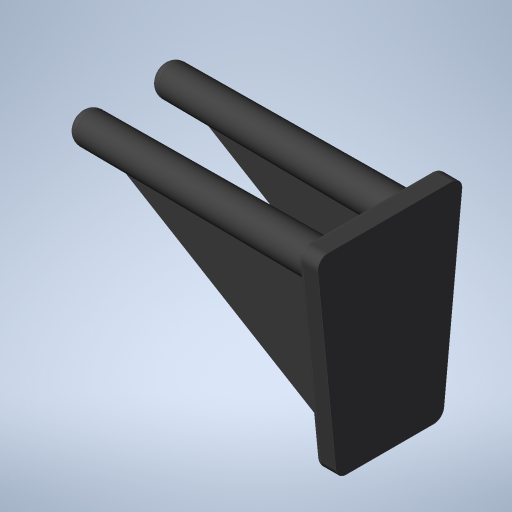
# Autodesk Inventor part: Ski Rack
Saved by Autodesk Inventor 2023 (Build 270158000, 158)
## iProperties
Created: 2022-12-21
Part Number: Ski Rack
Material: Generic
Document SubType Name: Modeling
Designer: tommy
Density: 1 g/cm^3
Appearance: Default
Author: tommy
Autodesk Inventor part; units mm, degrees
ref_plane "YZ Plane" through (0, 0, 0) normal (1, 0, 0) x (0, 1, 0)
ref_plane "XZ Plane" through (0, 0, 0) normal (0, 1, 0) x (-1, 0, 0)
ref_plane "XY Plane" through (0, 0, 0) normal (0, 0, 1) x (1, 0, 0)
sketch "Sketch3" plane through (0, 0, 0) normal (1, 0, 0) x (0, 1, 0)
  line L0 (-85.725, 0) -> (-85.725, -1.5875)
  line L1 (-85.725, -1.5875) -> (-85.725, 1.5875)
  line L2 (-85.725, 1.5875) -> (-9.3918, 1.5875)
  line L3 (-85.725, -1.5875) -> (-9.3918, -1.5875)
  line L4 (-85.725, -50.8) -> (-85.725, -49.2125)
  line L5 (-85.725, -49.2125) -> (-85.725, -52.3875)
  line L6 (-85.725, -52.3875) -> (-9.3918, -52.3875)
  line L7 (-85.725, -49.2125) -> (-9.3918, -49.2125)
  circle A0 centre (0, 0) radius 9.525
  circle A1 centre (0, -50.8) radius 9.525
  line L8 (-98.425, 1.5875) -> (12.7, 12.7)
  line L9 (-98.425, -52.3875) -> (12.7, -63.5)
  line L10 (12.7, 12.7) -> (12.7, -63.5)
  line L11 (-98.425, -52.3875) -> (-98.425, 1.5875)
  line L12 (19.05, -70.5167) -> (-104.775, -58.1342)
  line L13 (-104.775, -58.1342) -> (-104.775, 7.3342)
  line L14 (-104.775, 7.3342) -> (19.05, 19.7167)
  line L15 (19.05, 19.7167) -> (19.05, -70.5167)
  dimension "d14" = 1.5875
  dimension "d15" = 3.175
  dimension "d40" = 6.35
  constraints: 32 end point, 2 coincident, 2 parallel, 2 point on line, 1 perpendicular, 1 vertical, 9 other
  measures "d14" distance of L0.start L0.end
  measures "d15" distance of L0.end L1.end
  measures "d40" distance between parallel lines of L10 L15
extrude "Extrusion2" add sketch "Sketch3" along normal blind 12.7 contours L1 L2 A0 L3 L0 | A0 | L4 L7 A1 L6 L5 | A1 | L8 L10 L9 L11 | L12 L13 L14 L15
extrude "Extrusion3" add sketch "Sketch3" against normal blind 152.4 contours A0 | A1
extrude "Extrusion4" add sketch "Sketch3" against normal blind 127 contours L1 L2 A0 L3 L0 | L4 L7 A1 L6 L5
sketch "Sketch4" plane through (-127, -9.3918, 1.5875) normal (0, 0, 1) x (1, 0, 0)
  line L0 (0, -0.1332) -> (-25.4, -0.1332) projected
  line L1 (127, -76.3332) -> (0, -76.3332) projected
  line L2 (0, -0.1332) -> (127, -76.3332)
  line L3 (127, -76.3332) -> (0, -76.3332)
  line L4 (0, 0) -> (0, -0.1332) projected
  line L5 (0, -76.3332) -> (0, -0.1332)
  point P0 (127, 9.3918)
  constraints: 6 end point, 1 collinear, 1 perpendicular, 1 point on line
extrude "Extrusion5" cut sketch "Sketch4" against normal blind 127
draft "FaceDraft2" angle 0.4 pull direction (-1, 0, 0) faces at (-93.1333, -8.9299, 3.314) fixed edges at (-127, -9.4916, -0.7965) (-127, -9.4916, 0.7965)
draft "FaceDraft3" angle 0.4 pull direction (-1, 0, 0) faces at (-93.1333, -8.9299, -47.486) fixed edges at (-127, -9.4916, -51.5965) (-127, -9.4916, -50.0035)
fillet "Fillet3" radius 6.35 2 edges at (-152.4, -9.3477, 0) (-152.4, -9.3477, -50.8)
fillet "Fillet5" radius 6.35 4 edges at (6.35, 19.05, -70.5167) (6.35, 19.05, 19.7167) (6.35, -104.775, -58.1342) (6.35, -104.775, 7.3342)
fillet "Fillet6" radius 3.175 9 edges at (0, -103.1332, 5.8484) (0, -104.775, -25.4) (0, -103.1332, -56.6484) (0, -36.8284, -64.9288) (0, -92.3909, -59.3726) (0, 16.9609, -68.2082) (0, 19.05, -25.4) (0, 16.9609, 17.4082) (0, -43.4943, 13.4622)
chamfer "Chamfer1" distance 1.0583 angle 45 8 edges at (0, 0.7961, -40.4188) (0, 0.7961, -61.1812) (0, -48.0075, -52.3875) (0, 0.7961, 10.3812) (0, 0.7961, -10.3812) (0, -48.0075, -1.5875) (0, -48.0075, -49.2125) (0, -48.0075, 1.5875)
body "Solid2"
